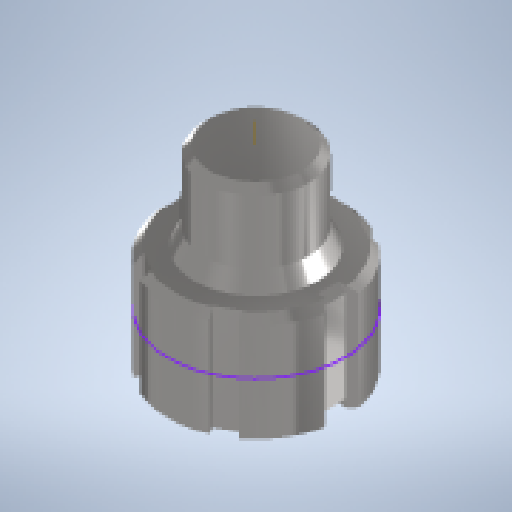
# Autodesk Inventor part: base_hydraulic_pump
Saved by Autodesk Inventor 2023 (Build 270158000, 158)
## iProperties
Created: 2023-11-19
Part Number: base_hydraulic_pump
Material: Stainless Steel
Document SubType Name: Modeling
Designer: Beatrice
Density: 8 g/cm^3
Appearance: Semi-Polished
Author: Beatrice
Autodesk Inventor part; units mm, degrees
ref_plane "YZ Plane" through (0, 0, 0) normal (1, 0, 0) x (0, 1, 0)
ref_plane "XZ Plane" through (0, 0, 0) normal (0, 1, 0) x (-1, 0, 0)
ref_plane "XY Plane" through (0, 0, 0) normal (0, 0, 1) x (1, 0, 0)
sketch "Sketch1" plane through (0, 0, 0) normal (0, 0, 1) x (1, 0, 0)
  circle A0 centre (0, 0) radius 15
  circle A1 centre (0, 0) radius 25
  dimension "d0" = 30
  constraints: 2 centre point, 2 coincident
  measures "d0" diameter of A0
extrude "Extrusion1" add sketch "Sketch1" along normal mid plane 30
extrude "Extrusion2" add sketch "Sketch1" against normal blind 10 contours A0
extrude "Extrusion3" add sketch "Sketch1" along normal blind 40 contours A0
chamfer "Chamfer1" distance 2 angle 45 1 edges at (-25, 0, 15)
sketch "Sketch2" plane through (0, 0, -15) normal (0, 0, -1) x (-1, 0, 0)
  circle A0 centre (0, 0) radius 25 projected
  circle A1 centre (0, 0) radius 15 projected
  line L0 (-22.5, 3) -> (-25.5, 3)
  line L1 (-25.5, 3) -> (-25.5, -3)
  line L2 (-25.5, -3) -> (-22.5, -3)
  line L3 (-22.5, -3) -> (-22.5, 3)
  line L4 (-22.5, 3) -> (-25.5, -3) construction
  line L5 (-25.5, 3) -> (-22.5, -3) construction
  point P0 (-24, 0)
  dimension "d12" = 6
  dimension "d13" = 24
  dimension "d14" = 3
  constraints: 12 end point, 2 midpoint, 2 parallel, 1 horizontal, 1 horizontal alignment, 1 perpendicular
  measures "d12" distance of L0.end L1.end
  measures "d13" distance of point (-24, 0) point (0, 0)
  measures "d14" distance between parallel lines of L3 L1
extrude "Extrusion4" cut sketch "Sketch2" against normal through all contours L0 L3 L2 A0 | A0 L2 L1 L0 picked at (-23.3266, 0.334)
chamfer "Chamfer2" distance 2 angle 45 5 edges at (24.8193, -3, -1) (24.8193, 3, -1) (22.5, 0, -15) (22.5, 0, 15) (-15, 0, 40)
pattern_circular "Circular Pattern1" count 6 over 360 about axis through (0, 0, -10) along (0, 0, 1) of "Extrusion4"
sketch "Sketch3" plane through (0, 0, 15) normal (0, 0, 1) x (1, 0, 0)
  circle A0 centre (0, 0) radius 15 projected
  line L0 (20.5, 3) -> (20.5, -3) projected
  line L1 (20.5, -3) -> (22.8035, -3) projected
  arc A1 (13.9998, -18.2484) -> (22.8035, -3) centre (0, 0) ccw projected
  line L2 (13.9998, -18.2484) -> (13.8481, -17.9856) projected
  line L3 (13.8481, -17.9856) -> (8.6519, -20.9856) projected
  line L4 (8.6519, -20.9856) -> (8.8037, -21.2484) projected
  arc A2 (-8.8037, -21.2484) -> (8.8037, -21.2484) centre (0, 0) ccw projected
  line L5 (-8.8037, -21.2484) -> (-8.6519, -20.9856) projected
  line L6 (-8.6519, -20.9856) -> (-13.8481, -17.9856) projected
  line L7 (-13.8481, -17.9856) -> (-13.9998, -18.2484) projected
  arc A3 (-22.8035, -3) -> (-13.9998, -18.2484) centre (0, 0) ccw projected
  line L8 (-22.8035, -3) -> (-22.5, -3) projected
  line L9 (-22.5, -3) -> (-22.5, 3) projected
  line L10 (-22.5, 3) -> (-22.8035, 3) projected
  arc A4 (-13.9998, 18.2484) -> (-22.8035, 3) centre (0, 0) ccw projected
  line L11 (-13.9998, 18.2484) -> (-13.8481, 17.9856) projected
  line L12 (-13.8481, 17.9856) -> (-8.6519, 20.9856) projected
  line L13 (-8.6519, 20.9856) -> (-8.8037, 21.2484) projected
  arc A5 (8.8037, 21.2484) -> (-8.8037, 21.2484) centre (0, 0) ccw projected
  line L14 (8.8037, 21.2484) -> (8.6519, 20.9856) projected
  line L15 (8.6519, 20.9856) -> (13.8481, 17.9856) projected
  line L16 (13.8481, 17.9856) -> (13.9998, 18.2484) projected
  arc A6 (22.8035, 3) -> (13.9998, 18.2484) centre (0, 0) ccw projected
  line L17 (22.8035, 3) -> (20.5, 3) projected
  circle A7 centre (0, 0) radius 17.5
  dimension "d21" = 35
  constraints: 1 centre point, 1 coincident
  measures "d21" diameter of A7
extrude "Extrusion5" add sketch "Sketch3" along normal blind 5 contours A7
sketch "Sketch4" plane through (0, 0, 0) normal (1, 0, 0) x (0, 1, 0)
  line L0 (15, 20) -> (-15, 20) projected
  line L1 (15, 38) -> (-15, 38) projected
  line L2 (17.5, 20) -> (-17.5, 20) projected
  line L3 (-17.5, 15) -> (17.5, 15) projected
  line L4 (-19.9942, 13) -> (-19.9942, -15) projected
  line L5 (-4.9744, -15) -> (-19.9942, -15) projected
  line L6 (-4.9744, 13) -> (-4.9744, -15) projected
  line L7 (-19.9942, 13) -> (-4.9744, 13) projected
  line L8 (-15, 20) -> (-17.5, 15)
  line L9 (-18.2484, 15) -> (-3, 15) projected
  line L10 (-15, 15) -> (-15, 20)
  line L11 (-17.5, 15) -> (-15, 15)
  line L12 (-15, 20) -> (-17.5, 20)
  line L13 (-17.5, 20) -> (-17.5, 15)
  line L14 (-17.5, 15) -> (-15, 15)
  line L15 (-15, 15) -> (-15, 20)
  line L16 (0, -26) -> (0, 51) projected
  point P0 (0, 0)
  constraints: 14 end point, 2 parallel, 2 perpendicular, 1 collinear, 1 horizontal, 1 point on line
revolve "Revolution1" cut sketch "Sketch4" angle 360 about axis through (0, 0, -10) along (0, 0, 1) contours L8 L13 L2
body "Solid1"
